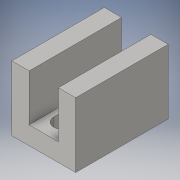
# Autodesk Inventor part: frame_mount
Saved by Autodesk Inventor 2016 (Build 200138000, 138)
## iProperties
Created: 2016-03-06
Part Number: frame_mount
Material: Generic
Document SubType Name: Modeling
Designer: dimas
Density: 1 g/cm^3
Appearance: Default
Author: dimas
Autodesk Inventor part; units mm, degrees
ref_plane "YZ Plane" through (0, 0, 0) normal (1, 0, 0) x (0, 1, 0)
ref_plane "XZ Plane" through (0, 0, 0) normal (0, 1, 0) x (-1, 0, 0)
ref_plane "XY Plane" through (0, 0, 0) normal (0, 0, 1) x (1, 0, 0)
sketch "Sketch1" plane through (0, 0, 0) normal (0, 1, 0) x (-1, 0, 0)
  line L0 (0, 0) -> (17.526, 0)
  line L1 (17.526, 0) -> (17.526, 25.4)
  line L2 (17.526, 25.4) -> (0, 25.4)
  line L3 (0, 25.4) -> (0, 0)
  dimension "d0" = 17.526
  dimension "d1" = 25.4
  constraints: 8 end point, 2 parallel, 1 horizontal, 1 perpendicular
  measures "d0" distance of L2.end L1.end
  measures "d1" distance of L1.end L0.end
extrude "Extrusion1" add sketch "Sketch1" along normal blind 17.78
sketch "Sketch2" plane through (0, 17.78, 0) normal (0, 1, 0) x (1, 0, 0)
  line L0 (0, -25.4) -> (0, 0) projected
  line L1 (0, 0) -> (-4.7498, 0)
  line L2 (0, 0) -> (-17.526, 0) projected
  line L3 (-17.526, 0) -> (-12.7762, 0)
  line L4 (-12.7762, 0) -> (-4.7498, 0)
  line L5 (-4.7498, 0) -> (-4.7498, -25.4)
  line L6 (-4.7498, -25.4) -> (-12.7762, -25.4)
  line L7 (-12.7762, -25.4) -> (-12.7762, 0)
  dimension "d4" = 4.7498
  dimension "d5" = 4.7498
  constraints: 12 end point, 2 parallel, 2 point on line, 1 horizontal, 1 perpendicular
  measures "d4" distance of L0.end L1.end
  measures "d5" distance of L2.end L3.end
extrude "Extrusion2" cut sketch "Sketch2" against normal blind 12.827
sketch "Sketch5" plane through (0, 4.953, 0) normal (0, 1, 0) x (1, 0, 0)
  line L0 (-17.526, -25.4) -> (0, -25.4) projected
  line L1 (-8.763, -25.4) -> (-8.763, -20.066)
  line L2 (-8.763, -25.4) -> (-8.763, -10.0584)
  line L3 (-8.763, -10.0584) -> (-8.763, -7.5184)
  circle A0 centre (-8.763, -7.5184) radius 2.54
  circle A1 centre (-8.763, -20.066) radius 2.54
  line L4 (-6.223, -7.5184) -> (-6.223, -20.066)
  line L5 (-11.303, -7.5184) -> (-11.303, -20.066)
  point P0 (0, 0)
  dimension "d14" = 5.334
  dimension "d15" = 15.3416
  dimension "d16" = 2.54
  dimension "d17" = 5.08
  dimension "d18" = 5.08
  constraints: 10 end point, 4 point on circle, 2 centre point, 2 coincident, 2 tangent, 2 vertical, 1 midpoint, 1 perpendicular
  measures "d14" distance of L1.start L1.end
  measures "d15" distance of L1.start L2.end
  measures "d16" distance of L2.end L3.end
  measures "d17" diameter of A0
  measures "d18" diameter of A1
extrude "Extrusion3" cut sketch "Sketch5" against normal blind 12.827
body "Solid1"
